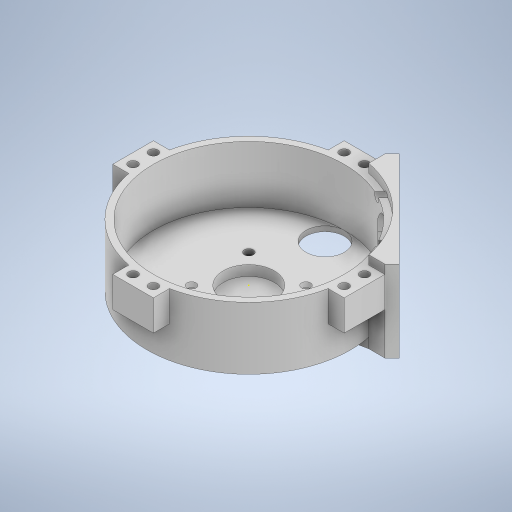
# Autodesk Inventor part: CO-0-01-ArmMotorMount
Saved by Autodesk Inventor 2023 (Build 270158000, 158)
## iProperties
Created: 2023-09-27
Part Number: CO-0-01-ArmMotorMount
Material: Generic
Document SubType Name: Modeling
Designer: thesl
Density: 1 g/cm^3
Appearance: Default
Mass: 82.7387 g
Surface Area: 399.617 cm^2
Volume: 82.7387 cm^3
Author: thesl
Autodesk Inventor part; units mm, degrees
ref_plane "YZ Plane" through (0, 0, 0) normal (1, 0, 0) x (0, 1, 0)
ref_plane "XZ Plane" through (0, 0, 0) normal (0, 1, 0) x (-1, 0, 0)
ref_plane "XY Plane" through (0, 0, 0) normal (0, 0, 1) x (1, 0, 0)
sketch "Sketch1" plane through (0, 0, 0) normal (0, 1, 0) x (-1, 0, 0)
  circle A0 centre (0, 0) radius 50.8
  dimension "d0" = 101.6
  constraints: 1 centre point, 1 coincident
  measures "d0" diameter of A0
extrude "Extrusion1" add sketch "Sketch1" along normal blind 34.925
sketch "Sketch2" plane through (0, 34.925, 0) normal (0, 1, 0) x (1, 0, 0)
  circle A0 centre (0, 0) radius 47.625
  dimension "d3" = 95.25
  constraints: 1 centre point, 1 coincident
  measures "d3" diameter of A0
extrude "Extrusion2" cut sketch "Sketch2" against normal blind 32.385
sketch "Sketch3" plane through (0, 2.54, 0) normal (0, 1, 0) x (1, 0, 0)
  circle A0 centre (0, 0) radius 12.7
  dimension "d6" = 25.4
  constraints: 1 centre point, 1 coincident
  measures "d6" diameter of A0
extrude "Extrusion3" cut sketch "Sketch3" against normal blind 28.575
sketch "Sketch4" plane through (0, 2.54, 0) normal (0, 1, 0) x (1, 0, 0)
  line L0 (14.2875, -14.2875) -> (-14.2875, -14.2875)
  line L1 (-14.2875, -14.2875) -> (-14.2875, 14.2875)
  line L2 (-14.2875, 14.2875) -> (14.2875, 14.2875)
  line L3 (14.2875, 14.2875) -> (14.2875, -14.2875)
  line L4 (14.2875, -14.2875) -> (-14.2875, 14.2875) construction
  line L5 (-14.2875, -14.2875) -> (14.2875, 14.2875) construction
  point P0 (0, 0)
  dimension "d9" = 28.575
  dimension "d10" = 28.575
  constraints: 12 end point, 2 midpoint, 2 parallel, 1 horizontal, 1 perpendicular
  measures "d9" distance of L0.start L0.end
  measures "d10" distance of L0.end L1.end
hole "Hole1" at (-14.2875, 2.54, 14.2875) at (-14.2875, 2.54, -14.2875) at (14.2875, 2.54, -14.2875) at (14.2875, 2.54, 14.2875) direction (0, -1, 0) diameter 4.4958 end through all clearance for "Flat Head Machine Screw (82)" size "#8" standard "Ansi Unified Screw Threads"
sketch "Sketch5" plane through (0, 34.925, 0) normal (0, 1, 0) x (1, 0, 0)
  circle A0 centre (0, 0) radius 47.625 projected
  line L0 (0, -47.625) -> (-10.16, -47.625)
  line L1 (-10.16, -47.625) -> (-10.16, -57.785)
  line L2 (-10.16, -57.785) -> (0, -57.785)
  line L3 (0, -57.785) -> (0, -47.625)
  line L4 (0, -47.625) -> (10.16, -47.625)
  line L5 (10.16, -47.625) -> (10.16, -57.785)
  line L6 (10.16, -57.785) -> (0, -57.785)
  line L7 (0, -57.785) -> (0, -47.625)
  dimension "d18" = 10.16
  dimension "d19" = 10.16
  dimension "d20" = 10.16
  dimension "d21" = 10.16
  constraints: 16 end point, 4 parallel, 2 horizontal, 2 perpendicular, 1 vertical alignment, 1 other
  measures "d18" distance of L2.end L1.end
  measures "d19" distance of L0.end L1.end
  measures "d20" distance of L5.end L6.end
  measures "d21" distance of L4.end L5.end
extrude "Extrusion4" add sketch "Sketch5" against normal blind 19.05 contours L4 L5 L6 L3 | L3 L2 L1 L0
sketch "Sketch6" plane through (0, 34.925, 0) normal (0, 1, 0) x (1, 0, 0)
  circle A0 centre (0, 0) radius 47.625 projected
  line L0 (-47.625, 0) -> (-57.785, 0)
  line L1 (-57.785, 0) -> (-57.785, 10.16)
  line L2 (-57.785, 10.16) -> (-47.625, 10.16)
  line L3 (-47.625, 10.16) -> (-47.625, -10.16)
  line L4 (-47.625, -10.16) -> (-57.785, -10.16)
  line L5 (-57.785, -10.16) -> (-57.785, 0)
  line L6 (0, 47.626) -> (10.16, 47.626)
  line L7 (10.16, 47.626) -> (10.16, 57.786)
  line L8 (10.16, 57.786) -> (-10.16, 57.786)
  line L9 (-10.16, 57.786) -> (-10.16, 47.626)
  line L10 (-10.16, 47.626) -> (0, 47.626)
  line L11 (47.625, 0) -> (57.785, 0)
  line L12 (57.785, 0) -> (57.785, 10.16)
  line L13 (57.785, 10.16) -> (47.625, 10.16)
  line L14 (47.625, 10.16) -> (47.625, -10.16)
  line L15 (47.625, -10.16) -> (57.785, -10.16)
  line L16 (57.785, -10.16) -> (57.785, 0)
  dimension "d24" = 10.16
  dimension "d25" = 10.16
  dimension "d26" = 20.32
  dimension "d27" = 10.16
  dimension "d28" = 10.16
  dimension "d29" = 20.32
  dimension "d30" = 10.16
  dimension "d31" = 10.16
  dimension "d32" = 20.32
  constraints: 34 end point, 14 perpendicular, 3 horizontal, 3 point on line, 2 point on circle
  measures "d24" distance of L0.start L0.end
  measures "d25" distance of L0.end L1.end
  measures "d26" distance of L2.end L3.end
  measures "d27" distance of L6.start L6.end
  measures "d28" distance of L6.end L7.end
  measures "d29" distance of L7.end L8.end
  measures "d30" distance of L11.start L11.end
  measures "d31" distance of L11.end L12.end
  measures "d32" distance of L13.end L14.end
extrude "Extrusion5" add sketch "Sketch6" against normal blind 19.05 contours L3 L4 L5 L0 | L0 L1 L2 L3 | L10 L9 L8 L7 L6 | L14 L13 L12 L11 | L11 L16 L15 L14
sketch "Sketch7" plane through (0, 34.925, 0) normal (0, 1, 0) x (1, 0, 0)
  line L0 (-10.16, 57.786) -> (10.16, 57.786) projected
  line L1 (0, 57.786) -> (0, 52.706)
  line L2 (0, 52.706) -> (-5.08, 52.706)
  line L3 (-10.16, 49.7736) -> (-10.16, 57.786) projected
  line L4 (-5.08, 52.706) -> (5.08, 52.706)
  line L5 (57.785, 10.16) -> (57.785, -10.16) projected
  line L6 (57.785, 0) -> (52.705, 0)
  line L7 (52.705, 0) -> (52.705, 5.08)
  line L8 (52.705, 5.08) -> (52.705, -5.08)
  line L9 (-10.16, -57.785) -> (10.16, -57.785) projected
  line L10 (0, -57.785) -> (0, -52.705)
  line L11 (0, -52.705) -> (5.08, -52.705)
  line L12 (5.08, -52.705) -> (-5.08, -52.705)
  line L13 (-57.785, -10.16) -> (-57.785, 10.16) projected
  line L14 (-57.785, 0) -> (-52.705, 0)
  line L15 (-52.705, 0) -> (-52.705, 5.08)
  line L16 (-52.705, 5.08) -> (-52.705, -5.08)
  point P0 (0, 0)
  dimension "d35" = 5.08
  dimension "d36" = 5.08
  dimension "d37" = 10.16
  dimension "d38" = 5.08
  dimension "d39" = 5.08
  dimension "d40" = 10.16
  dimension "d41" = 5.08
  dimension "d42" = 5.08
  dimension "d43" = 5.08
  dimension "d44" = 5.08
  dimension "d45" = 10.16
  constraints: 24 end point, 4 midpoint, 4 perpendicular, 4 point on line, 2 horizontal, 2 vertical
  measures "d35" distance of L1.start L1.end
  measures "d36" distance of L1.end L2.end
  measures "d37" distance of L2.end L4.end
  measures "d38" distance of L6.start L6.end
  measures "d39" distance of L6.end L7.end
  measures "d40" distance of L7.end L8.end
  measures "d41" distance of L10.start L10.end
  measures "d42" distance of L10.end L11.end
  measures "d43" distance of L14.start L14.end
  measures "d44" distance of L14.end L15.end
  measures "d45" distance of L15.end L16.end
hole "Hole2" at (-5.08, 34.925, -52.706) at (5.08, 34.925, -52.706) at (52.705, 34.925, -5.08) at (52.705, 34.925, 5.08) at (5.08, 34.925, 52.705) at (-5.08, 34.925, 52.705) at (-52.705, 34.925, 5.08) at (-52.705, 34.925, -5.08) direction (0, -1, 0) diameter 4.4958 depth 19.05 tip angle 118 clearance for "Flat Head Machine Screw (82)" size "#8" standard "Ansi Unified Screw Threads"
sketch "Sketch8" plane through (0, 2.54, 0) normal (0, 1, 0) x (1, 0, 0)
  line L0 (0, 0) -> (0, 38.1)
  circle A0 centre (0, 38.1) radius 9.525
  dimension "d53" = 38.1
  constraints: 2 end point, 1 centre point, 1 coincident, 1 vertical
  measures "d53" distance of L0.start L0.end
extrude "Extrusion6" cut sketch "Sketch8" against normal blind 19.05
sketch "Sketch10" plane through (0, 2.54, 0) normal (0, 1, 0) x (1, 0, 0)
  point P0 (0, 0)
sketch "Sketch11" plane through (0, 34.925, 0) normal (0, 1, 0) x (1, 0, 0)
  circle A0 centre (0, 0) radius 72.1958
  constraints: 1 centre point, 1 coincident
extrude "Extrusion7" cut sketch "Sketch11" against normal blind 3.81
sketch "Sketch12" plane through (0, 0, 0) normal (0, -1, 0) x (1, 0, 0)
  circle A0 centre (0, 0) radius 12.7 projected
  circle A1 centre (0, 0) radius 25.4
  circle A2 centre (0, 0) radius 12.7
  circle A3 centre (14.2875, -14.2875) radius 2.2479 projected
  circle A4 centre (14.2875, -14.2875) radius 3.4925
  circle A5 centre (-14.2875, -14.2875) radius 2.2479 projected
  circle A6 centre (-14.2875, -14.2875) radius 3.4925
  circle A7 centre (-14.2875, 14.2875) radius 2.2479 projected
  circle A8 centre (-14.2875, 14.2875) radius 3.4925
  circle A9 centre (14.2875, 14.2875) radius 2.2479 projected
  circle A10 centre (14.2875, 14.2875) radius 3.4925
  dimension "d68" = 50.8
  dimension "d69" = 6.985
  dimension "d70" = 6.985
  dimension "d71" = 6.985
  dimension "d72" = 6.985
  constraints: 6 centre point, 6 coincident
  measures "d68" diameter of A1
  measures "d69" diameter of A4
  measures "d70" diameter of A6
  measures "d71" diameter of A8
  measures "d72" diameter of A10
extrude "Extrusion8" add sketch "Sketch12" along normal blind 2.54 contours A1
sketch "Sketch13" plane through (0, -2.54, 0) normal (0, -1, 0) x (1, 0, 0)
  circle A0 centre (0, 0) radius 25.4
  circle A1 centre (14.2875, 14.2875) radius 2.2479 projected
  circle A2 centre (14.2875, 14.2875) radius 3.4925
  circle A3 centre (14.2875, -14.2875) radius 2.2479 projected
  circle A4 centre (14.2875, -14.2875) radius 3.4925
  circle A5 centre (-14.311, -14.2875) radius 3.4926
  circle A6 centre (-14.2875, 14.2875) radius 3.4925
  constraints: 5 centre point, 3 coincident
extrude "Extrusion9" add sketch "Sketch13" along normal blind 2.54 contours A0
sketch "Sketch17" plane through (0, 31.115, 0) normal (0, 1, 0) x (1, 0, 0)
  line L0 (57.785, 10.16) -> (57.785, -10.16) projected
  line L1 (10.16, 57.786) -> (10.16, 49.7736) projected
  line L2 (10.16, 57.786) -> (10.16, 49.7736)
  line L3 (10.16, 49.7736) -> (22.304, 45.6418)
  arc A0 (49.7736, 10.16) -> (10.16, 49.7736) centre (0, 0) ccw projected
  line L4 (57.785, 10.16) -> (49.7736, 10.16)
  line L5 (49.7736, 10.16) -> (45.6512, 22.2941)
  line L6 (57.785, 10.16) -> (45.6423, 22.303)
  line L7 (22.304, 45.6418) -> (10.16, 57.786)
  point P0 (45.6617, 22.2633)
  constraints: 12 end point, 2 point on circle, 1 collinear, 1 point on line
extrude "Extrusion11" add sketch "Sketch17" along normal blind 4.445 and the other way blind 36.195 contours L7 A0 L1 | A0 L3 | A0 L5 L6 L4
sketch "Sketch18" plane through (0, 31.115, 0) normal (0, 1, 0) x (1, 0, 0)
  line L0 (57.785, 10.16) -> (57.785, -10.16) projected
  line L1 (10.16, 57.786) -> (10.16, 49.7736) projected
  line L2 (57.785, 10.16) -> (10.16, 57.786)
  line L3 (10.16, 57.786) -> (13.7521, 61.3781)
  line L4 (13.7521, 61.3781) -> (61.3771, 13.7521)
  line L5 (61.3771, 13.7521) -> (57.785, 10.16)
  point P0 (0, 0)
  dimension "d81" = 5.08
  constraints: 8 end point, 3 perpendicular, 1 point on line
  measures "d81" distance of L1.start L3.end
extrude "Extrusion12" add sketch "Sketch18" along normal blind 4.445 and the other way blind 36.195
sketch "Sketch19" plane through (0, 0, 0) normal (0, -1, 0) x (1, 0, 0)
  line L0 (10.16, -57.786) -> (10.16, -49.7736) projected
  line L1 (49.7736, -10.16) -> (57.785, -10.16) projected
  arc A0 (10.16, -49.7736) -> (49.7736, -10.16) centre (0, 0) ccw
  line L2 (0, 0) -> (49.7736, -10.16)
  line L3 (0, 0) -> (2.0739, -10.16)
  circle A1 centre (0, -38.1) radius 9.525 projected
  arc A2 (8.609, -42.1755) -> (6.323, -30.9765) centre (0, -38.1) ccw
  line L4 (0, 0) -> (6.323, -30.9765)
  line L5 (8.609, -42.1755) -> (10.16, -49.7736)
  circle A3 centre (14.2875, -14.2875) radius 2.2479 projected
  circle A4 centre (14.2875, -14.2875) radius 2.2479
  circle A5 centre (14.2875, -14.2875) radius 3.4925
  point P0 (0, -47.625)
  point P1 (6.323, -30.9765)
  point P2 (8.609, -42.1755)
  constraints: 8 end point, 5 point on circle, 4 centre point, 4 coincident, 1 point on line, 1 other
extrude "Extrusion13" add sketch "Sketch19" along normal blind 5.08 contours L5 A1 L4 L3 L2 A0
sketch "Sketch20" plane through (0, -2.54, 0) normal (0, 1, 0) x (1, 0, 0)
  line L0 (12.4434, 2.54) -> (0, 0) projected
  circle A0 centre (0, 0) radius 12.7
  constraints: 1 centre point, 1 coincident
extrude "Extrusion14" cut sketch "Sketch20" along normal blind 27.6225
sketch "Sketch23" plane through (0, 31.115, 0) normal (0, 1, 0) x (1, 0, 0)
  arc A0 (10.16, 49.7736) -> (49.7736, 10.16) centre (0, 0) ccw projected
  line L0 (0, 0) -> (10.16, 49.7736)
  line L1 (0, 0) -> (49.7736, 10.16)
  line L2 (57.785, 10.16) -> (49.7736, 10.16) projected
  arc A1 (49.7736, 10.16) -> (10.16, 49.7736) centre (0, 0) ccw
  constraints: 4 end point, 2 point on circle, 1 centre point, 1 coincident
extrude "Extrusion16" cut sketch "Sketch23" along normal blind 7.62 contours A1 L1 L0
sketch "Sketch24" plane through (13.7521, -5.08, -61.3781) normal (0.7071143, 0, -0.7070992) x (-0.7070992, 0, -0.7071143)
  line L0 (-67.3526, 40.64) -> (0, 40.64) projected
  line L1 (-67.3526, 40.64) -> (-67.3526, 20.32)
  line L2 (-67.3526, 20.32) -> (-33.6722, 20.32)
  line L3 (0, 0) -> (0, 20.955) projected
  line L4 (-48.6582, 5.334) -> (-18.6862, 5.334)
  line L5 (-18.6862, 5.334) -> (-18.6862, 35.306)
  line L6 (-18.6862, 35.306) -> (-48.6582, 35.306)
  line L7 (-48.6582, 35.306) -> (-48.6582, 5.334)
  line L8 (-48.6582, 5.334) -> (-18.6862, 35.306) construction
  line L9 (-18.6862, 5.334) -> (-48.6582, 35.306) construction
  point P0 (-33.6772, 5.08)
  dimension "d107" = 20.32
  dimension "d108" = 33.6804
  dimension "d109" = 29.972
  dimension "d110" = 29.972
  constraints: 16 end point, 2 midpoint, 2 parallel, 2 perpendicular, 1 vertical
  measures "d107" distance of L0.start L1.end
  measures "d108" distance of L1.end L2.end
  measures "d109" distance of L4.start L4.end
  measures "d110" distance of L5.end L4.end
hole "Hole5" at (48.1583, 30.226, -26.9711) at (26.9652, 30.226, -48.1648) at (26.9652, 0.254, -48.1648) at (48.1583, 0.254, -26.9711) direction (-0.7071143, 0, 0.7070992) diameter 4.2926 depth 19.05 tip angle 118 clearance for "Socket Head Cap Screw" size "M4" standard "Ansi Metric M Profile"
sketch "Sketch25" plane through (13.7521, -5.08, -61.3781) normal (0.7071143, 0, -0.7070992) x (-0.7070992, 0, -0.7071143)
  line L0 (-67.3526, 0) -> (-67.3526, 40.64) projected
  line L1 (-67.3526, 40.64) -> (-67.3526, 20.32)
  line L2 (-33.6772, 20.32) -> (-33.6772, 5.08)
  line L3 (-48.9172, 29.845) -> (-48.9172, 10.795)
  line L4 (-48.9172, 10.795) -> (-18.4372, 10.795)
  line L5 (-18.4372, 10.795) -> (-18.4372, 29.845)
  line L6 (-18.4372, 29.845) -> (-48.9172, 29.845)
  line L7 (-48.9172, 29.845) -> (-18.4372, 10.795) construction
  line L8 (-48.9172, 10.795) -> (-18.4372, 29.845) construction
  arc A0 (-18.4372, 20.32) -> (-48.9172, 20.32) centre (-33.6772, 20.32) ccw
  dimension "d118" = 19.05
  dimension "d119" = 30.48
  constraints: 16 end point, 5 midpoint, 2 parallel, 2 point on circle, 1 centre point, 1 coincident, 1 perpendicular, 1 vertical
  measures "d118" distance of L3.start L3.end
  measures "d119" distance of L4.end L3.end
extrude "Extrusion17" cut sketch "Sketch25" against normal blind 7.62 contours A0 L6 L5 L4 L3 | A0 L6
body "Solid1"
